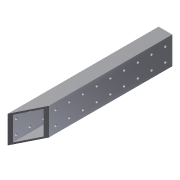
# Autodesk Inventor part: Frame_MidRollerSupport
Saved by Autodesk Inventor 2012 (Build 160160000, 160)
## iProperties
Created: 2012-01-09
Part Number: Frame_MidRollerSupport
Material: Default
Document SubType Name: Modeling
Designer: JesseK
Density: 1 g/cm^3
Mass: 110.399 g
Surface Area: 728.78 cm^2
Volume: 110.399 cm^3
Author: JesseK
Autodesk Inventor part; units mm, degrees
ref_plane "YZ Plane" through (0, 0, 0) normal (1, 0, 0) x (0, 1, 0)
ref_plane "XZ Plane" through (0, 0, 0) normal (0, 1, 0) x (-1, 0, 0)
ref_plane "XY Plane" through (0, 0, 0) normal (0, 0, 1) x (1, 0, 0)
sketch "Sketch1" plane through (0, 0, 0) normal (0, 0, 1) x (1, 0, 0)
  line L0 (0, 0) -> (25.4, 0)
  line L1 (25.4, 0) -> (25.4, 50.8)
  line L2 (25.4, 50.8) -> (0, 50.8)
  line L3 (0, 50.8) -> (0, 0)
  dimension "d0" = 25.4
  dimension "d1" = 50.8
  constraints: 8 end point, 2 parallel, 1 horizontal, 1 perpendicular
  measures "d0" distance of L1.end L2.end
  measures "d1" distance of L0.end L1.end
extrude "Extrusion1" add sketch "Sketch1" along normal blind 279.4
shell "Shell1" thickness 3.175 removed faces 2 at (8.4667, 33.8667, 0) at (8.4667, 33.8667, 279.4)
sketch "Sketch2" plane through (25.4, 0, 0) normal (1, 0, 0) x (0, 0, -1)
  line L0 (-279.4, 50.8) -> (-279.4, 0) projected
  line L1 (0, 50.8) -> (-279.4, 50.8) projected
  circle A0 centre (-266.7, 38.1) radius 2.3813
  dimension "d5" = 4.7625
  dimension "d6" = 12.7
  dimension "d7" = 12.7
  constraints: 1 centre point
  measures "d5" diameter of A0
  measures "d6" distance from line of L1 A0.centre
  measures "d7" distance from line of L0 A0.centre
extrude "Extrusion2" cut sketch "Sketch2" against normal through all
pattern_linear "Rectangular Pattern1" count 11 spacing 25.4 along (0, 0, -1) count 2 spacing 25.4 along (0, -1, 0) of "Extrusion2"
sketch "Sketch3" plane through (0, 50.8, 0) normal (0, 1, 0) x (1, 0, 0)
  line L0 (0, -279.4) -> (25.4, -279.4) projected
  line L1 (25.4, 0) -> (25.4, -279.4) projected
  line L2 (0, -279.4) -> (25.4, -279.4)
  line L3 (25.4, -228.6) -> (0, -279.4)
  dimension "d16" = 50.8
  constraints: 4 end point, 1 collinear, 1 point on line
  measures "d16" distance of L0.end L3.start
extrude "Extrusion3" cut sketch "Sketch3" against normal through all
body "Solid1"
